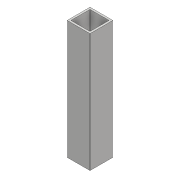
# Autodesk Inventor part: WeldingDemo
Saved by Autodesk Inventor 2017 (Build 210142000, 142)
## iProperties
Created: 2017-03-29
Part Number: WeldingDemo
Material: Generic
Document SubType Name: Modeling
Designer: krosie
Density: 1 g/cm^3
Appearance: Default
Author: krosie
Autodesk Inventor part; units mm, degrees
ref_plane "YZ Plane" through (0, 0, 0) normal (1, 0, 0) x (0, 1, 0)
ref_plane "XZ Plane" through (0, 0, 0) normal (0, 1, 0) x (-1, 0, 0)
ref_plane "XY Plane" through (0, 0, 0) normal (0, 0, 1) x (1, 0, 0)
sketch "Sketch1" plane through (0, 0, 0) normal (0, 0, 1) x (1, 0, 0)
  line L0 (-9.3, -9.5) -> (9.3, -9.5)
  line L1 (9.5, -9.3) -> (9.5, 9.3)
  line L2 (9.3, 9.5) -> (-9.3, 9.5)
  line L3 (-9.5, 9.3) -> (-9.5, -9.3)
  line L4 (-9.5, -9.5) -> (9.5, 9.5) construction
  line L5 (9.5, -9.5) -> (-9.5, 9.5) construction
  line L6 (-7.7, 7.9) -> (7.7, 7.9)
  line L7 (7.9, 7.7) -> (7.9, -7.7)
  line L8 (7.7, -7.9) -> (-7.7, -7.9)
  line L9 (-7.9, -7.7) -> (-7.9, 7.7)
  arc A0 (-7.7, 7.9) -> (-7.9, 7.7) centre (-7.7, 7.7) ccw
  arc A1 (-7.9, -7.7) -> (-7.7, -7.9) centre (-7.7, -7.7) ccw
  arc A2 (7.7, -7.9) -> (7.9, -7.7) centre (7.7, -7.7) ccw
  arc A3 (7.9, 7.7) -> (7.7, 7.9) centre (7.7, 7.7) ccw
  arc A4 (-9.3, 9.5) -> (-9.5, 9.3) centre (-9.3, 9.3) ccw
  arc A5 (-9.5, -9.3) -> (-9.3, -9.5) centre (-9.3, -9.3) ccw
  arc A6 (9.3, -9.5) -> (9.5, -9.3) centre (9.3, -9.3) ccw
  arc A7 (9.5, 9.3) -> (9.3, 9.5) centre (9.3, 9.3) ccw
  point P0 (0, 0)
  dimension "d0" = 19
  dimension "d1" = 19
  dimension "d2" = 1.6
  dimension "d3" = 0.2
  dimension "d4" = 0.2
  dimension "d5" = 0.2
  dimension "d6" = 0.2
  dimension "d7" = 0.2
  dimension "d8" = 0.2
  dimension "d9" = 0.2
  dimension "d10" = 0.2
  constraints: 20 end point, 16 point on circle, 16 tangent, 8 centre point, 8 point on line, 4 parallel, 2 midpoint, 2 perpendicular, 1 horizontal, 3 other
  measures "d0" distance of L5.end L4.end
  measures "d1" distance of L5.start L4.end
  measures "d2" distance between parallel lines of L2 L6
  measures "d3" radius of A0
  measures "d4" radius of A1
  measures "d5" radius of A2
  measures "d6" radius of A3
  measures "d7" radius of A4
  measures "d8" radius of A5
  measures "d9" radius of A6
  measures "d10" radius of A7
extrude "Extrusion1" add sketch "Sketch1" along normal blind 100
sketch "Sketch2" plane through (9.5, -9.3, 0) normal (1, 0, 0) x (0, 0, -1)
  line L0 (0, 17.2) -> (-1.6, 18.8)
  line L1 (0, 18.8) -> (-100, 18.8) projected
  line L2 (0, 17.2) -> (2.2627, 17.2) construction
  line L3 (-1.6, 18.8) -> (0, 18.8)
  line L4 (0, 18.8) -> (0, 17.2)
  line L5 (0, 1.4) -> (-100, 1.4) projected
  line L6 (0, 1.4) -> (-1.6, -0.2)
  line L7 (0, -0.2) -> (-100, -0.2) projected
  line L8 (0, 1.4) -> (2.2627, 1.4) construction
  line L9 (-1.6, -0.2) -> (0, -0.2)
  line L10 (0, -0.2) -> (0, 1.4)
  line L11 (0, 0) -> (0, 18.6) projected
  point P0 (0, 9.3)
  dimension "d13" = 135
  dimension "d14" = 135
  constraints: 16 end point, 3 collinear, 2 equal length, 2 horizontal, 2 point on line, 1 perpendicular
  measures "d13" angle of L2 L0
  measures "d14" angle of L6 L8
extrude "Extrusion2" cut sketch "Sketch2" against normal through all
sketch "Sketch3" plane through (-9.3, 9.5, 100) normal (0, 1, 0) x (1, 0, 0)
  line L0 (1.3863, 100) -> (16.0747, 100) construction
  line L1 (-0.2, 98.6) -> (-0.2, 0) projected
  line L2 (18.8, 98.6) -> (18.8, 0) projected
  line L3 (1.4, 100) -> (-0.2, 98.4)
  line L4 (1.4, 100) -> (3.6627, 100) construction
  line L5 (-0.2, 98.4) -> (-0.2, 100)
  line L6 (-0.2, 100) -> (1.4, 100)
  line L7 (17.2, 100) -> (18.8, 98.4)
  line L8 (17.2, 100) -> (19.4627, 100) construction
  line L9 (18.8, 98.4) -> (18.8, 100)
  line L10 (18.8, 100) -> (17.2, 100)
  point P0 (9.3, 100)
  dimension "d18" = 135
  dimension "d19" = 45
  constraints: 18 end point, 5 point on line, 3 horizontal, 2 equal length, 2 perpendicular
  measures "d18" angle of L3 L4
  measures "d19" angle of L7 L8
extrude "Extrusion3" cut sketch "Sketch3" against normal through all
body "Solid1"
